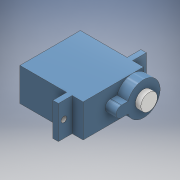
# Autodesk Inventor part: learnbotServo
Saved by Autodesk Inventor 2017 (Build 210142000, 142)
## iProperties
Part Number: learnbotServo
Material: Genérico
Document SubType Name: Modeling
Designer: rober
Density: 1 g/cm^3
Appearance: Valor por defecto
Author: rober
Autodesk Inventor part; units mm, degrees
ref_plane "YZ Plane" through (0, 0, 0) normal (1, 0, 0) x (0, 1, 0)
ref_plane "XZ Plane" through (0, 0, 0) normal (0, 1, 0) x (-1, 0, 0)
ref_plane "XY Plane" through (0, 0, 0) normal (0, 0, 1) x (1, 0, 0)
sketch "Boceto1" plane through (0, 0, 0) normal (0, 0, 1) x (1, 0, 0)
  line L0 (0, 2.4) -> (0, 0.2)
  line L1 (0, 0.2) -> (1.7, 0.2)
  line L2 (0, 2.4) -> (1.7, 2.4)
  line L3 (1.7, 2.4) -> (1.7, 2.9)
  line L4 (1.7, 2.9) -> (1.9, 2.9)
  line L5 (1.9, 2.9) -> (1.9, 2.4)
  line L6 (1.9, 2.4) -> (2.3, 2.4)
  line L7 (2.3, 2.4) -> (2.3, 0.2)
  line L8 (2.3, 2.4) -> (2.7, 2.4)
  line L9 (2.7, 1.2) -> (2.7, 0.8)
  line L10 (2.7, 0.8) -> (2.3, 0.8)
  line L11 (1.7, 0.2) -> (1.7, -0.3)
  line L12 (1.7, -0.3) -> (1.9, -0.3)
  line L13 (1.9, -0.3) -> (1.9, 0.2)
  line L14 (1.9, 0.2) -> (2.3, 0.2)
  line L15 (2.3, 1.2) -> (2.7, 1.2)
  line L16 (2.7, 1.2) -> (2.7, 2.4)
  line L17 (2.7, 1.5) -> (2.9, 1.5)
  line L18 (2.9, 1.5) -> (2.9, 2.1)
  line L19 (2.9, 2.1) -> (2.7, 2.1)
  line L20 (2.3, 0.2) -> (3.3416, 0.2)
  point P0 (0, 0)
  constraints: 42 end point, 4 point on line
extrude "Extrusión1" add sketch "Boceto1" along normal blind 1.2 contours L2 L3 L4 L5 L6 L7 L14 L13 L12 L11 L1 L0
sketch "Boceto2" plane through (2.3, 0.2, 0) normal (1, 0, 0) x (0, 0, -1)
  line L0 (0, 0) -> (0, 2.2) projected
  line L1 (0, 2.2) -> (-1.2, 2.2) projected
  line L2 (-1.2, 0) -> (-1.2, 2.2) projected
  line L3 (-1.2, 2.4) -> (-1.2, 0)
  line L4 (-1.2, 0) -> (0, 0)
  line L5 (0, 2.4) -> (-1.2, 2.4)
  line L6 (-1.2, 2.9) -> (0, 2.9)
  line L7 (-1.2, 2.9) -> (-1.2, 2.4)
  line L8 (-1.2, -0.5) -> (0, -0.5)
  line L9 (0, -0.5) -> (0, 2.9)
  line L10 (-1.2, 0) -> (-1.2, -0.5)
  arc A0 (-0.4, 1.2343) -> (-0.8, 1.2343) centre (-0.6, 1.8) ccw
  circle A1 centre (-0.6, 1.8) radius 0.3
  arc A2 (-0.8, 1) -> (-0.4, 1) centre (-0.6, 1) ccw
  line L11 (-0.8, 1) -> (-0.8, 1.2343)
  line L12 (-0.4, 1) -> (-0.4, 1.2343)
  line L13 (0, 0) -> (-1.2, 0) projected
  point P0 (0, -0.2)
  constraints: 20 end point, 4 point on circle, 3 centre point, 2 point on line
extrude "Extrusión2" add sketch "Boceto2" along normal blind 0.4 contours A0 L12 A2 L11 L1 | L1 A0 | A1
sketch "Boceto3" plane through (2.7, 0.2, 0) normal (1, 0, 0) x (0, 0, -1)
  line L0 (-1.2, 2.4) -> (-1.2, 0)
  line L1 (-1.2, 0) -> (0, 0)
  line L2 (0, 2.4) -> (-1.2, 2.4)
  line L3 (-1.2, 2.9) -> (0, 2.9)
  line L4 (-1.2, 2.9) -> (-1.2, 2.4)
  line L5 (-1.2, -0.5) -> (0, -0.5)
  line L6 (0, -0.5) -> (0, 2.9)
  line L7 (-1.2, 0) -> (-1.2, -0.5)
  arc A0 (-0.4, 1.2343) -> (-0.8, 1.2343) centre (-0.6, 1.8) ccw
  circle A1 centre (-0.6, 1.8) radius 0.3
  arc A2 (-0.8, 1) -> (-0.4, 1) centre (-0.6, 1) ccw
  line L8 (-0.8, 1) -> (-0.8, 1.2343)
  line L9 (-0.4, 1) -> (-0.4, 1.2343)
  arc A3 (-0.4, 1.2343) -> (-0.8, 1.2343) centre (-0.6, 1.8) ccw projected
  line L10 (-0.8, 1.2343) -> (-0.8, 1) projected
  arc A4 (-0.8, 1) -> (-0.4, 1) centre (-0.6, 1) ccw projected
  line L11 (-0.4, 1) -> (-0.4, 1.2343) projected
  point P0 (0, -0.2)
  constraints: 20 end point, 4 point on circle, 3 centre point, 2 point on line
extrude "Extrusión3" add sketch "Boceto3" along normal blind 0.2 contours A1
sketch "Boceto6" plane through (1.9, -0.3, 0) normal (1, 0, 0) x (0, 0, -1)
  line L0 (0, 0) -> (-1.2, 0) projected
  circle A0 centre (-0.6, 0.2) radius 0.1
  line L1 (0, 3.2) -> (-1.2, 3.2) projected
  circle A1 centre (-0.6, 3) radius 0.1
  point P0 (0, 0.3)
  constraints: 2 centre point
extrude "Extrusión4" cut sketch "Boceto6" against normal blind 10
